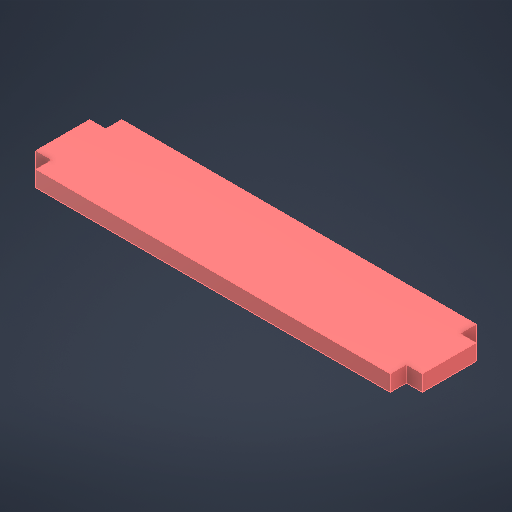
# Autodesk Inventor part: support
Saved by Autodesk Inventor 2025.3 (Build 293356030, 356C)
## iProperties
Created: 2025-09-04
Part Number: support
Material: 木材 (楓木)
Document SubType Name: Modeling
Designer: 陳泓任
Density: 0.67 g/cm^3
Appearance: 平滑 - 紅色
Author: 陳泓任
Autodesk Inventor part; units mm, degrees
ref_plane "YZ Plane" through (0, 0, 0) normal (1, 0, 0) x (0, 1, 0)
ref_plane "XZ Plane" through (0, 0, 0) normal (0, 1, 0) x (-1, 0, 0)
ref_plane "XY Plane" through (0, 0, 0) normal (0, 0, 1) x (1, 0, 0)
sketch "草圖1" plane through (0, 0, 0) normal (0, 1, 0) x (-1, 0, 0)
  line L0 (0, 5) -> (3, 5)
  line L1 (3, 5) -> (3, 8)
  line L2 (69, 5) -> (69, 8)
  line L3 (69, 5) -> (72, 5)
  line L4 (69, -5) -> (72, -5)
  line L5 (69, -5) -> (69, -8)
  line L6 (3, -5) -> (3, -8)
  line L7 (0, -5) -> (3, -5)
  line L8 (3, -8) -> (69, -8)
  line L9 (72, -5) -> (72, 5)
  line L10 (69, 8) -> (3, 8)
  line L11 (0, 5) -> (0, -5)
  line L12 (0, 0) -> (0, -38.3248)
  dimension "d0" = 66
  dimension "d1" = 10
  dimension "d2" = 3
  dimension "d3" = 3
  dimension "d5" = 72
  constraints: 26 end point, 5 collinear, 5 equal length, 2 parallel, 1 coincident, 1 midpoint, 1 perpendicular, 1 vertical
  measures "d0" distance of L2.end L1.end
  measures "d1" distance of L4.end L3.end
  measures "d2" distance of L0.end L1.end
  measures "d3" distance of L0.start L0.end
  measures "d5" distance between parallel lines of L11 L9
extrude "擠出1" add sketch "草圖1" along normal blind 3
